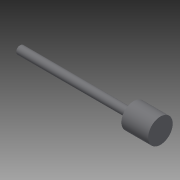
# Autodesk Inventor part: D-95381.5-0.25XP-3.356-3pos
Saved by Autodesk Inventor 2014 (Build 180170000, 170)
## iProperties
Created: 2014-01-19
Part Number: D-95381.5-0.25XP-3.356-3pos
Material: Generic
Catalog Web Link: www.cadenas.de
Description: 3 Pos Rod Cyl-Original Line Cyl
Vendor: BIMBA
Document SubType Name: Standard Catalog Part
Designer: Michael
Manufacturer: BIMBA
Density: 1 g/cm^3
Appearance: RGB(180.00000447034725,180.00000447034725,180.00000447034725)
Category: PARTsolutions
Company: BIMBA
Title: D-95381.5-0.25XP-3.356-3pos
Author: Cadenas PARTsolutions
Comments: Original Line Cyl
PSOL_IDENT_0: {$CADENAS_DATA\23d-libs\bimba\bimba\bimba_imperial\bimba_full_line\original_line_cylinders\three_pos
PSOL_IDENT_1: ition_cylinders\3pos_rod.prj},236 {VTYP=3D},{NB=D-95381.5-0.25XP-3.356-3pos},{LINA=D-95381.5-0.25XP-
PSOL_IDENT_2: 3.356-3pos},{NN=3 Pos Rod Cyl},{DATE=16.11.2011 06:17:30},{GEOMDATE=16.11.2011 00:00:00},{VERSION=},
PSOL_IDENT_3: {LINEID=60},{LINESUBID=-1},{WBVAR=STROKEA,STROKEB,MNT,BUMPER,Q,L,NT}  {NB=D-95381.5-0.25XP-3.356-3po
PSOL_IDENT_4: s},{LINA=D-95381.5-0.25XP-3.356-3pos},{KT=DUMMY},{PN=D-9538},{GROOVE=0.00000000},{START=0.50000000},
PSOL_IDENT_5: {I=0},{PNN=1},{LL=2},{STROKEA=1.500},{STROKEB=0.250},{MNT=XP},{BUMPER=},{Q=},{L=3.356},{NT=},{NDL=0.
PSOL_IDENT_6: 19000000},{NDL1=0.19000000},{NDDL=0},{NDDL1=0.00000000},{NDLL=0.00000000},{NDR=0.19000000},{NDDR=0.3
PSOL_IDENT_7: 7500000},{NDRR=0.00000000},{WF=0.00000000},{WFW=0.00000000},{WFL=0.00000000},{LMIN=0.998},{DRAW=3},{
PSOL_IDENT_8: CHL=0.00000000},{CL=0.00000000},{WL=0.00000000},{RL=0.00000000},{CHR=0.20000000},{CR=0.14050000},{WR=
PSOL_IDENT_9: 0.04950000},{RR=0.01850000},{D=0.00000000},{DD=0.00000000},{CH=0.00000000},{R=0.00000000},{LLRR=0.00
PSOL_IDENT_10: 100000},{LL1B1=0.06000000},{LL1B2=0.00000000},{LL1B3=0.00000000},{LL1B4=0.00000000},{LL1B=0},{LL1R1=
PSOL_IDENT_11: 0.07700000},{LL1R2=0.07700000},{LL1R3=0.01100000},{LL1R4=0.01000000},{LL1R=0.077},{ADDERWBB=0.000000
PSOL_IDENT_12: 00},{ADDERWBA=0.00000000},{ADDERWBBXP=0.00000000},{ADDERWBAXP=0.00000000},{ADDERBB=0.00000000},{ADDE
PSOL_IDENT_13: RBA=0.00000000},{ADDERBBXP=0.00000000},{ADDERBAXP=0.00000000},{B=0.57300000},{A7=0.13200000},{ADD1=0
PSOL_IDENT_14: .00200000},{ADD2=0.00200000},{ADD11=-0.00200000},{ADD22=0.00400000},{ADDER=0.13300000},{A8=0.0250000
PSOL_IDENT_15: 0},{H1=0.15700000},{H2=0.15600000},{RH=0.157},{CENL=0.158},{CENR=0.158},{RG=0.15700000},{DIMBBL=1.00
PSOL_IDENT_16: 000000},{DIMABL=0.93800000},{BBL=1.06200000},{ABL=1.06200000},{STROKEALGA=[0.001:31.989/0.001]},{STR
PSOL_IDENT_17: OKEALGB=[0.001:30.5/0.001]},{STROKEBMAX=30.500},{BLB=2.750},{BLA=2.438},{LLL=0.685},{LLR=0.623}
CNS_NN: 3 Pos Rod Cyl
CNS_NT: Standard
CNS_NB: D-95381.5-0.25XP-3.356-3pos
CNS_NBSYN: $PN.$STROKEA.-$STROKEB.$MNT.$BUMPER.$Q.$NT.-$L.-3pos
CNS_LINA: D-95381.5-0.25XP-3.356-3pos
CNS_PN: D-9538
CNS_GROOVE: 0.00000000
CNS_START: 0.50000000
CNS_I: 0
CNS_PNN: 1
CNS_LL: 2
CNS_STROKEA: 1.500
CNS_STROKEB: 0.250
CNS_MNT: Universal Mounting
CNS_BUMPER: w/o Bumper
CNS_Q: Without Side Ported Rear Head
CNS_L: 3.356
CNS_NDL: 0.19000000
CNS_NDL1: 0.19000000
CNS_NDDL: 0.000
CNS_NDDL1: 0.00000000
CNS_NDLL: 0.00000000
CNS_NDR: 0.19000000
CNS_NDDR: 0.37500000
CNS_NDRR: 0.00000000
CNS_WF: 0.00000000
CNS_WFW: 0.00000000
CNS_WFL: 0.00000000
CNS_LMIN: 0.998
CNS_DRAW: 3
CNS_CHL: 0.00000000
CNS_CL: 0.00000000
CNS_WL: 0.00000000
CNS_RL: 0.00000000
CNS_CHR: 0.20000000
CNS_CR: 0.14050000
CNS_WR: 0.04950000
CNS_RR: 0.01850000
CNS_D: 0.00000000
CNS_DD: 0.00000000
CNS_CH: 0.00000000
CNS_R: 0.00000000
CNS_LLRR: 0.00100000
CNS_LL1B1: 0.06000000
CNS_LL1B2: 0.00000000
CNS_LL1B3: 0.00000000
CNS_LL1B4: 0.00000000
CNS_LL1B: 0.000
CNS_LL1R1: 0.07700000
CNS_LL1R2: 0.07700000
CNS_LL1R3: 0.01100000
CNS_LL1R4: 0.01000000
CNS_LL1R: 0.077
CNS_ADDERWBB: 0.00000000
CNS_ADDERWBA: 0.00000000
CNS_ADDERWBBXP: 0.00000000
CNS_ADDERWBAXP: 0.00000000
CNS_ADDERBB: 0.00000000
CNS_ADDERBA: 0.00000000
CNS_ADDERBBXP: 0.00000000
CNS_ADDERBAXP: 0.00000000
CNS_B: 0.57300000
CNS_A7: 0.13200000
CNS_ADD1: 0.00200000
CNS_ADD2: 0.00200000
CNS_ADD11: -0.00200000
CNS_ADD22: 0.00400000
CNS_ADDER: 0.13300000
CNS_A8: 0.02500000
CNS_H1: 0.15700000
CNS_H2: 0.15600000
CNS_RH: 0.157
CNS_CENL: 0.158
CNS_CENR: 0.158
CNS_RG: 0.15700000
CNS_DIMBBL: 1.00000000
CNS_DIMABL: 0.93800000
CNS_BBL: 1.06200000
CNS_ABL: 1.06200000
CNS_STROKEALGA: [0.001:31.989/0.001]
CNS_STROKEALGB: [0.001:30.5/0.001]
CNS_STROKEBMAX: 30.500
CNS_BLB: 2.750
CNS_BLA: 2.438
CNS_LLL: 0.685
CNS_LLR: 0.623
SUPPLIER: BIMBA
ARTICLENO: D-95381.5-0.25XP-3.356-3pos
BOMINFO: D-95381.5-0.25XP-3.356-3pos
CREATOR: CADENAS GmbH
Autodesk Inventor part; units mm, degrees
ref_plane "YZ Plane" through (0, 0, 0) normal (1, 0, 0) x (0, 1, 0)
ref_plane "XZ Plane" through (0, 0, 0) normal (0, 1, 0) x (-1, 0, 0)
ref_plane "XY Plane" through (0, 0, 0) normal (0, 0, 1) x (1, 0, 0)
sketch "Sketch_5" plane through (0, 0, 0) normal (0, 0, 1) x (1, 0, 0)
  line L0 (-9.525, 0) -> (-85.2424, 0)
  line L1 (-85.2424, 0) -> (-85.2424, 1.9406)
  line L2 (-85.2424, 1.9406) -> (-84.77, 2.413)
  line L3 (-84.77, 2.413) -> (-9.525, 2.413)
  line L4 (-9.525, 2.413) -> (-9.525, 0)
  line L5 (-9.525, 0) -> (-85.2424, 0)
  constraints: 12 end point
revolve "Revolution1" add sketch "Sketch_5" angle 360 about axis through (-9.525, 0, 0) along (1, 0, 0)
sketch "Sketch_14" plane through (0, 0, 0) normal (0, 0, 1) x (1, 0, 0)
  line L0 (-1.9558, 0) -> (-17.78, 0)
  line L1 (-17.78, 0) -> (-17.78, 7.2771)
  line L2 (-17.78, 7.2771) -> (-1.9558, 7.2771)
  line L3 (-1.9558, 7.2771) -> (-1.9558, 0)
  line L4 (-1.9558, 0) -> (-17.78, 0)
  constraints: 10 end point
revolve "Revolution2" add sketch "Sketch_14" angle 360 about axis through (-1.9558, 0, 0) along (1, 0, 0)
ref_plane "h1_XY" through (-85.2424, 0, 0) normal (0, 1, 0) x (1, 0, 0)
ref_plane "h1_YZ" through (-85.2424, 0, 0) normal (1, 0, 0) x (0, 0, -1)
ref_plane "h1_ZX" through (-85.2424, 0, 0) normal (0, 0, -1) x (0, 1, 0)
ref_plane "h2_XY" through (-85.2424, 0, 0) normal (0, 1, 0) x (1, 0, 0)
ref_plane "h2_YZ" through (-85.2424, 0, 0) normal (1, 0, 0) x (0, 0, -1)
ref_plane "h2_ZX" through (-85.2424, 0, 0) normal (0, 0, -1) x (0, 1, 0)
ref_plane "k1_XY" through (-85.2424, 0, -2.413) normal (0, 1, 0) x (1, 0, 0)
ref_plane "k1_YZ" through (-85.2424, 0, -2.413) normal (1, 0, 0) x (0, 0, -1)
ref_plane "k1_ZX" through (-85.2424, 0, -2.413) normal (0, 0, -1) x (0, 1, 0)
ref_plane "k2_XY" through (-85.2424, 0, 2.413) normal (0, 1, 0) x (1, 0, 0)
ref_plane "k2_YZ" through (-85.2424, 0, 2.413) normal (1, 0, 0) x (0, 0, -1)
ref_plane "k2_ZX" through (-85.2424, 0, 2.413) normal (0, 0, -1) x (0, 1, 0)
ref_plane "start_XY" through (-72.5424, 0, 0) normal (0, 1, 0) x (1, 0, 0)
ref_plane "start_YZ" through (-72.5424, 0, 0) normal (1, 0, 0) x (0, 0, -1)
ref_plane "start_ZX" through (-72.5424, 0, 0) normal (0, 0, -1) x (0, 1, 0)
ref_plane "to_prc_XY" through (-85.2424, 0, 0) normal (1, 0, 0) x (0, 0, -1)
ref_plane "to_prc_YZ" through (-85.2424, 0, 0) normal (0, 0, -1) x (0, 1, 0)
ref_plane "to_prc_ZX" through (-85.2424, 0, 0) normal (0, 1, 0) x (1, 0, 0)
ref_plane "to_rod_guide_XY" through (-85.2424, 0, 0) normal (1, 0, 0) x (0, 0, -1)
ref_plane "to_rod_guide_YZ" through (-85.2424, 0, 0) normal (0, 0, -1) x (0, 1, 0)
ref_plane "to_rod_guide_ZX" through (-85.2424, 0, 0) normal (0, 1, 0) x (1, 0, 0)
body "Solid1"
